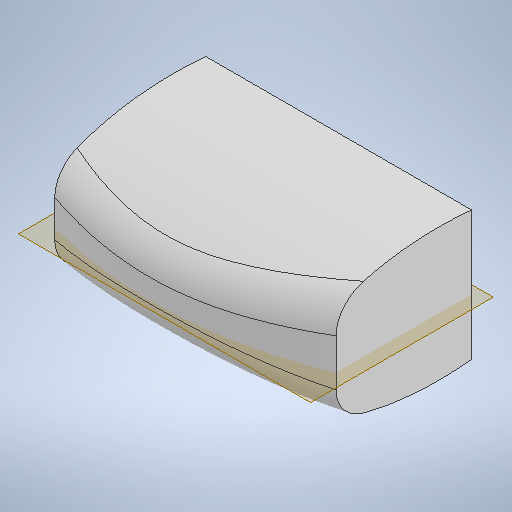
# Autodesk Inventor part: Body01
Saved by Autodesk Inventor 2025 (Build 290162000, 162)
## iProperties
Created: 2024-12-10
Part Number: Body01
Material: Generic
Document SubType Name: Modeling
Designer: naka6
Density: 1 g/cm^3
Appearance: Default
Author: naka6
Autodesk Inventor part; units mm, degrees
ref_plane "YZ Plane" through (0, 0, 0) normal (1, 0, 0) x (0, 1, 0)
ref_plane "XZ Plane" through (0, 0, 0) normal (0, 1, 0) x (-1, 0, 0)
ref_plane "XY Plane" through (0, 0, 0) normal (0, 0, 1) x (1, 0, 0)
sketch "スケッチ1" plane through (0, 0, 0) normal (0, 1, 0) x (-1, 0, 0)
  line L0 (-40, 25) -> (40, 25)
  line L1 (40, 25) -> (40, -25)
  line L2 (40, -25) -> (-40, -25)
  line L3 (-40, -25) -> (-40, 25)
  line L4 (-40, 25) -> (40, -25) construction
  line L5 (40, 25) -> (-40, -25) construction
  circle A0 centre (7, -100) radius 125
  line L6 (40, -15) -> (30, -25)
  point P0 (0, 0)
  point P1 (40, 20.5653)
  point P2 (-40, 15.8275)
  dimension "d0" = 80
  dimension "d1" = 50
  dimension "d2" = 7
  dimension "d3" = 250
  dimension "d6" = 10
  dimension "d7" = 10
  constraints: 14 end point, 2 midpoint, 2 parallel, 2 point on line, 1 centre point, 1 horizontal, 1 perpendicular, 1 tangent
  measures "d0" distance of L0.start L0.end
  measures "d1" distance of L2.end L0.start
  measures "d2" horizontal distance of A0.centre point (0, 0)
  measures "d3" diameter of A0
  measures "d6" distance of L1.end L6.end
  measures "d7" distance of L1.end L6.start
extrude "押し出し1" add sketch "スケッチ1" along normal blind 40 contours A0 L1 L6 L2 L3 | L1 L2 L6
ref_plane "作業平面1" through (0, 17.5, 0) normal (0, 1, 0) x (1, 0, 0)
sketch "スケッチ2" plane through (0, 17.5, 0) normal (0, 1, 0) x (1, 0, 0)
  line L0 (40, -15.8275) -> (40, 25) projected
  line L1 (40, 25) -> (-40, 25) projected
  line L2 (-40, 25) -> (-40, -20.5653) projected
  arc A0 (-40, -20.5653) -> (40, -15.8275) centre (-7, 100) ccw projected
  line L3 (-40, 15) -> (-30, 25)
  line L4 (40, 25) -> (-40, 25) projected
  point P0 (0, 0)
  dimension "d11" = 10
  dimension "d12" = 45
  constraints: 2 end point, 2 point on line
  measures "d11" distance from line of L1 L3.start
  measures "d12" angle of L2 L3
extrude "押し出し2" cut sketch "スケッチ2" along normal blind 5 contours L3 L2 L1
sketch "スケッチ3" plane through (40, 0, 15.8275) normal (1, 0, 0) x (0, 0, -1)
  line L0 (-9.1725, 0) -> (-9.1725, 40) projected
  line L1 (0, 0) -> (40.8275, 0) projected
  line L2 (0, 0) -> (-9.1725, 0) projected
  line L3 (0, 40) -> (-9.1725, 40) projected
  line L4 (0, 40) -> (40.8275, 40) projected
  line L5 (40.8275, 0) -> (40.8275, 40) projected
  line L6 (40.8275, 20) -> (-7.81, 20)
  ellipse E0 centre (30.8275, 20) end of major axis (-13.1725, 20) minor radius 20
  point P0 (15.8275, 0)
  point P1 (-4.7379, 0)
  point P2 (-4.7379, 40)
  point P3 (-9.1725, 28.332)
  point P4 (30.8275, 40)
  point P5 (40.8275, 39.4766)
  point P6 (30.8275, 0)
  point P7 (-9.1725, 11.668)
  point P8 (40.8275, 0.5234)
  dimension "d15" = 44
  dimension "d16" = 10
  constraints: 3 horizontal, 2 end point, 1 midpoint, 1 point on line, 2 other
  measures "d16" distance from line of L5 point (30.827, 20)
extrude "押し出し3" cut sketch "スケッチ3" against normal through all contours L0 E0 L1 L2 | L0 L3 L4 E0 | E0 L5 L1 | L4 L5 E0
fillet "フィレット2" radius 10 4 edges at (16.84, 9.6918, 22.7056) (-23.6437, 10.6425, 23.887) (16.84, 30.3082, 22.7056) (-23.6437, 29.3575, 23.887)
